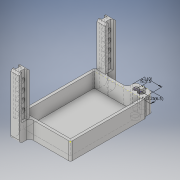
# Autodesk Inventor part: receiver_box_v1
Saved by Autodesk Inventor 2019 (Build 230136000, 136)
## iProperties
Created: 2020-04-16
Part Number: receiver_box_v1
Material: Generic
Document SubType Name: Modeling
Designer: close
Density: 1 g/cm^3
Appearance: Default
Author: close
Autodesk Inventor part; units mm, degrees
ref_plane "YZ Plane" through (0, 0, 0) normal (1, 0, 0) x (0, 1, 0)
ref_plane "XZ Plane" through (0, 0, 0) normal (0, 1, 0) x (-1, 0, 0)
ref_plane "XY Plane" through (0, 0, 0) normal (0, 0, 1) x (1, 0, 0)
sketch "Sketch1" plane through (0, 0, 0) normal (0, 1, 0) x (-1, 0, 0)
  line L0 (1, 0) -> (29, 0)
  line L1 (30, -1) -> (30, -42.75)
  line L2 (29, -43.75) -> (1, -43.75)
  line L3 (0, -42.75) -> (0, -1)
  arc A0 (30, -1) -> (29, 0) centre (29, -1) ccw
  arc A1 (1, 0) -> (0, -1) centre (1, -1) ccw
  arc A2 (0, -42.75) -> (1, -43.75) centre (1, -42.75) ccw
  arc A3 (29, -43.75) -> (30, -42.75) centre (29, -42.75) ccw
  point P0 (0, 0)
  point P1 (30, -43.75)
  point P2 (30, 0)
  point P3 (0, -43.75)
  dimension "d0" = 43.75
  dimension "d1" = 30
  dimension "d2" = 1
  constraints: 8 end point, 8 point on circle, 8 point on line, 8 tangent, 4 centre point, 3 equal radius, 2 parallel, 1 horizontal, 1 perpendicular
  measures "d0" distance of point (30, 0) point (30, -43.75)
  measures "d1" distance of point (30, -43.75) point (0, -43.75)
  measures "d2" radius of A0
extrude "Extrusion1" add sketch "Sketch1" along normal blind 10
shell "Shell1" thickness 1.5 removed faces 1 at (-20, 10, -14.9167)
sketch "Sketch2" plane through (0, 0, 0) normal (0, -1, 0) x (1, 0, 0)
  line L0 (-28.5, -49.75) -> (-28.5, 6) construction
  line L1 (-29, 0) -> (-1, 0) construction
  line L2 (-1, -43.75) -> (-29, -43.75) construction
  line L3 (-28.5, -49.75) -> (-23.6, -49.75)
  line L4 (-23.6, -49.75) -> (-23.6, -43.75)
  line L5 (-23.6, -43.75) -> (-28.5, -43.75)
  line L6 (-28.5, -43.75) -> (-28.5, -49.75)
  line L7 (-29, 0) -> (-1, 0) projected
  line L8 (-28.5, 6) -> (-23.6, 6)
  line L9 (-23.6, 6) -> (-23.6, 0)
  line L10 (-23.6, 0) -> (-28.5, 0)
  line L11 (-28.5, 0) -> (-28.5, 6)
  line L12 (-30, -42.75) -> (-30, -1) projected
  point P0 (0, 0)
  dimension "d6" = 55.75
  dimension "d7" = 43.75
  dimension "d8" = 6
  dimension "d9" = 4.9
  dimension "d10" = 1.5
  constraints: 18 end point, 4 parallel, 3 point on line, 2 horizontal, 2 perpendicular, 1 vertical
  measures "d6" distance of L0.start L0.end
  measures "d7" distance between parallel lines of L1 L2
  measures "d8" distance from line of L2 L0.start
  measures "d9" distance between parallel lines of L4 L0
  measures "d10" distance between parallel lines of L0 L12
extrude "Extrusion2" add sketch "Sketch2" against normal blind 35
fillet "Fillet1" radius 2 6 edges at (-28.5, 5, -43.75) (-28.5, 5, 0) (-23.6, 5, 0) (-26.05, 0, 6) (-26.05, 0, -49.75) (-23.6, 5, -43.75)
sketch "Sketch3" plane through (0, 0, 0) normal (0, -1, 0) x (1, 0, 0)
  circle A0 centre (-3.3527, -40.8144) radius 2.1095
  point P0 (0, 0)
  constraints: 1 centre point
extrude "Extrusion3" cut sketch "Sketch3" against normal up to surface (1.5 mm away)
sketch "Sketch4" plane through (0, 0, 0) normal (0, -1, 0) x (1, 0, 0)
  line L0 (-1, -43.75) -> (-21.6, -43.75) projected
  line L1 (-1, -43.75) -> (-11, -43.75)
  line L2 (-11, -43.75) -> (-11, -48.75)
  line L3 (-11, -48.75) -> (-1, -48.75)
  line L4 (-1, -48.75) -> (-1, -43.75)
  point P0 (0, 0)
  dimension "d16" = 5
  dimension "d17" = 10
  constraints: 8 end point, 2 parallel, 1 horizontal, 1 perpendicular
  measures "d16" distance between parallel lines of L0 L3
  measures "d17" distance between parallel lines of L4 L2
extrude "Extrusion4" add sketch "Sketch4" against normal blind 10
fillet "Fillet2" radius 2 4 edges at (-1, 5, -43.75) (-1, 5, -48.75) (-11, 5, -48.75) (-11, 5, -43.75)
sketch "Sketch5" plane through (0, 10, 0) normal (0, 1, 0) x (1, 0, 0)
  line L0 (-4.5, 45.5) -> (-7.5, 45.5) construction
  line L1 (-11, 46.75) -> (-11, 45.75) construction
  line L2 (-1, 44.9861) -> (-1, 46.75) construction
  line L3 (-3, 48.75) -> (-9, 48.75) construction
  line L4 (-28.5, 42.25) -> (-1.5, 42.25) construction
  point P0 (0, 0)
  dimension "d21" = 10
  dimension "d22" = 6.5
  dimension "d23" = 3.25
  dimension "d24" = 3
  dimension "d25" = 3.5
  constraints: 2 coincident, 2 end point, 1 horizontal
  measures "d21" distance between parallel lines of L1 L2
  measures "d22" distance between parallel lines of L3 L4
  measures "d23" distance between parallel lines of L4 L0
  measures "d24" distance of L0.start L0.end
  measures "d25" distance from line of L1 L0.end
hole "Hole1" at (-4.5, 10, -45.5) direction (0, -1, 0) diameter 3.5 end through all
hole "Hole2" at (-7.5, 10, -45.5) direction (0, -1, 0) diameter 2.85 end through all
sketch "Sketch6" plane through (0, 35, 0) normal (0, 1, 0) x (1, 0, 0)
  line L0 (-28.5, -1.575) -> (-27.25, -1.575)
  line L1 (-27.25, -1.575) -> (-27.25, -4.425)
  line L2 (-27.25, -4.425) -> (-28.5, -4.425)
  line L3 (-28.5, -4.425) -> (-28.5, -1.575)
  line L4 (-23.6, -4) -> (-23.6, -2) projected
  line L5 (-23.6, -1.575) -> (-24.85, -1.575)
  line L6 (-24.85, -1.575) -> (-24.85, -4.425)
  line L7 (-24.85, -4.425) -> (-23.6, -4.425)
  line L8 (-23.6, -4.425) -> (-23.6, -1.575)
  line L9 (-28.5, -6) -> (-23.6, -6) projected
  line L10 (-23.6, 0) -> (-28.5, 0) projected
  line L11 (-28.5, 48.175) -> (-27.25, 48.175)
  line L12 (-27.25, 48.175) -> (-27.25, 45.325)
  line L13 (-27.25, 45.325) -> (-28.5, 45.325)
  line L14 (-28.5, 45.325) -> (-28.5, 48.175)
  line L15 (-23.6, 48.175) -> (-24.85, 48.175)
  line L16 (-24.85, 48.175) -> (-24.85, 45.325)
  line L17 (-24.85, 45.325) -> (-23.6, 45.325)
  line L18 (-23.6, 45.325) -> (-23.6, 48.175)
  line L19 (-28.5, 43.75) -> (-23.6, 43.75) projected
  line L20 (-23.6, 49.75) -> (-28.5, 49.75) projected
  line L21 (-23.6, 43.75) -> (-23.6, 49.75) projected
  line L22 (-28.5, 49.75) -> (-28.5, 43.75) projected
  point P0 (0, 0)
  dimension "d44" = 2.85
  dimension "d45" = 6
  dimension "d46" = 1.575
  dimension "d47" = 2.85
  dimension "d48" = 6
  dimension "d49" = 1.575
  dimension "d50" = 2.4
  dimension "d51" = 4.9
  dimension "d52" = 1.25
  constraints: 32 end point, 8 parallel, 7 collinear, 4 horizontal, 4 perpendicular, 3 point on line
  measures "d44" distance between parallel lines of L2 L0
  measures "d45" distance between parallel lines of L9 L10
  measures "d46" distance between parallel lines of L9 L2
  measures "d47" distance of L11.end L12.end
  measures "d48" distance between parallel lines of L19 L20
  measures "d49" distance between parallel lines of L20 L11
  measures "d50" distance between parallel lines of L16 L12
  measures "d51" distance of L20.start L20.end
  measures "d52" distance between parallel lines of L21 L16
extrude "Extrusion5" cut sketch "Sketch6" against normal up to surface (25 mm away) contours L0 L1 L2 L3 | L8 L7 L6 L5 L4 | L11 L12 L13 L14 | L18 L17 L16 L15
chamfer "Chamfer1" distance 1 angle 45 4 edges at (-26.05, 35, 6) (-26.05, 35, 0) (-26.05, 35, -43.75) (-26.05, 35, -49.75)
sketch "Sketch7" plane through (-24.85, 35, 4.425) normal (1, 0, 0) x (0, 0, -1)
  line L0 (2.85, 0) -> (2.85, -25) projected
  line L1 (0, -25) -> (0, 0) projected
  line L2 (49.75, -25) -> (49.75, 0) projected
  line L3 (0, 0) -> (2.85, 0) projected
  point P0 (4.425, -35)
  point P1 (1.425, -5.35)
  point P2 (51.175, -5.35)
  point P3 (1.425, -10.35)
  point P4 (51.175, -10.35)
  point P5 (1.425, -15.35)
  point P6 (51.175, -15.35)
  point P7 (1.425, -20.35)
  point P8 (51.175, -20.35)
  dimension "d58" = 2.85
  dimension "d59" = 1.425
  dimension "d60" = 1.425
  dimension "d61" = 5.35
  dimension "d62" = 0
  dimension "d65" = 5
  constraints: 1 vertical, 6 other
  measures "d58" distance between parallel lines of L0 L1
  measures "d59" distance from line of L1 point (1.425, -5.35)
  measures "d60" distance from line of L2 point (51.175, -5.35)
  measures "d61" distance from line of L3 point (1.425, -5.35)
  measures "d62" vertical distance of point (1.425, -5.35) point (51.175, -5.35)
  measures "d65" distance of point (1.425, -5.35) point (1.425, -10.35)
hole "Hole3" at (-24.85, 29.65, 3) at (-24.85, 29.65, -46.75) at (-24.85, 24.65, 3) at (-24.85, 19.65, 3) at (-24.85, 14.65, 3) at (-24.85, 24.65, -46.75) at (-24.85, 19.65, -46.75) at (-24.85, 14.65, -46.75) direction (-1, 0, 0) diameter 2.75 end through all
equation "\"d8\" = -0.5 * d7 + 0.5 * d6"
equation "\"d23\" = 0.5 * d22"
equation "\"d25\" = -0.5 * d24 + 0.5 * d21"
equation "\"d44\" = d43"
equation "\"d46\" = -0.5 * d44 + 0.5 * d45"
equation "\"d49\" = -0.5 * d47 + 0.5 * d48"
equation "\"d52\" = -0.5 * d50 + 0.5 * d51"
equation "\"d59\" = 0.5 * d58"
equation "\"d60\" = d59"
equation "\"d43\" = 2.85"
body "Solid1"
